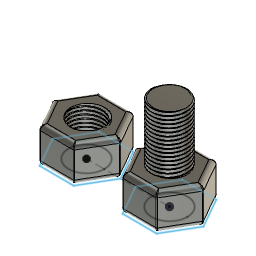
Nuts_and_Bolts (Autodesk Fusion 360 design; units mm, degrees)
Autodesk Fusion 360 part; units mm, degrees
sketch "Sketch1" plane through (0, 0, 0) normal (0, 0, 1) x (1, 0, 0)
sketch "Sketch3" plane through (0, 0, 0) normal (0, 0, 1) x (1, 0, 0)
  line L0 (7.3002, 12.4515) -> (-7.1332, 12.5479)
  line L1 (-7.1332, 12.5479) -> (-14.4334, 0.0964)
  line L2 (-14.4334, 0.0964) -> (-7.3002, -12.4515)
  line L3 (-7.3002, -12.4515) -> (7.1332, -12.5479)
  line L4 (7.1332, -12.5479) -> (14.4334, -0.0964)
  line L5 (14.4334, -0.0964) -> (7.3002, 12.4515)
  circle A0 centre (0, 0) radius 7.5
  line L6 (0, 0) -> (-35, 0) construction
  circle A1 centre (-35, 0) radius 7.5
  line L7 (-27.6998, 12.4515) -> (-42.1332, 12.5479)
  line L8 (-27.8668, -12.5479) -> (-20.5666, -0.0964)
  line L9 (-20.5666, -0.0964) -> (-27.6998, 12.4515)
  line L10 (-42.3002, -12.4515) -> (-27.8668, -12.5479)
  line L11 (-42.1332, 12.5479) -> (-49.4334, 0.0964)
  line L12 (-49.4334, 0.0964) -> (-42.3002, -12.4515)
  point P0 (-35, 0)
  point P1 (-35, 0)
  point P2 (-35, 0)
  dimension "d3" = 25
  dimension "d4" = 15
  dimension "d5" = 25
  dimension "d6" = 15
  dimension "d7" = 35
  constraint coincident A0.centre L6.start
  constraint horizontal L6
  constraint coincident P2 P1
  measures "d3" distance of L1.end L3.end
  measures "d4" diameter of A0
  measures "d5" distance of L11.end L8.start
  measures "d6" diameter of A1
  measures "d7" distance of A0.centre P2
sketch "Sketch4" plane through (0, 0, 0) normal (0, 0, 1) x (1, 0, 0)
extrude "Extrude1" add sketch "Sketch3" along normal blind 40 contours A0 makes body 1
extrude "Extrude2" add sketch "Sketch3" along normal blind 15 bodies 1 makes body 2 at (-27.5373, -0.7468, 10)
thread "Thread1" "ISO Metric profile 15.0 M15x1.5 6H" major diameter 15.2033 minor diameter 13.5262 pitch 1.5 angle 60 modelled right hand crest width 0.4068 on face at (-27.5373, -0.7468, 10) crest through (-28.2369, 0, 0.375) on bodies 2
thread "Thread2" "ISO Metric profile 15.0 M15x1.5 6g" major diameter 14.85 minor diameter 13.1369 pitch 1.5 angle 60 modelled right hand crest width 0.2152 on face at (7.4627, -0.7468, 23.3333) crest through (7.425, 0, 14.625) on bodies 1
fillet "Fillet1" radius 2 6 edges at (-0.0835, -12.4997, 15) (-10.8668, -6.1776, 15) (-10.7833, 6.3222, 15) (0.0835, 12.4997, 15) (10.8668, 6.1776, 15) (10.7833, -6.3222, 15) on bodies 1
fillet "Fillet2" radius 2 6 edges at (-24.2167, -6.3222, 15) (-35.0835, -12.4997, 15) (-45.8668, -6.1776, 15) (-45.7833, 6.3222, 15) (-34.9165, 12.4997, 15) (-24.1332, 6.1776, 15) on bodies 2
fillet "Fillet3" radius 2 12 edges at (0.0835, 12.4997, 0) (10.8668, 6.1776, 0) (10.7833, -6.3222, 0) (-0.0835, -12.4997, 0) (-10.8668, -6.1776, 0) (-10.7833, 6.3222, 0) (-34.9165, 12.4997, 0) (-24.1332, 6.1776, 0) (-24.2167, -6.3222, 0) (-35.0835, -12.4997, 0) (-45.8668, -6.1776, 0) (-45.7833, 6.3222, 0) on bodies 1 2
fillet "Fillet4" radius 0.5 36 edges at (6.799, -11.9599, 0.5858) (7.1332, -12.5479, 7.5) (6.799, -11.9599, 14.4142) (-6.9581, -11.868, 0.5858) (-7.3002, -12.4515, 7.5) (-6.9581, -11.868, 14.4142) (-13.757, 0.0919, 0.5858) (-14.4334, 0.0964, 7.5) (-13.757, 0.0919, 14.4142) (13.757, -0.0919, 0.5858) (14.4334, -0.0964, 7.5) (13.757, -0.0919, 14.4142) (6.9581, 11.868, 14.4142) (7.3002, 12.4515, 7.5) (6.9581, 11.868, 0.5858) (-6.799, 11.9599, 14.4142) (-7.1332, 12.5479, 7.5) (-6.799, 11.9599, 0.5858) (-28.0419, 11.868, 14.4142) (-27.6998, 12.4515, 7.5) (-28.0419, 11.868, 0.5858) (-41.799, 11.9599, 14.4142) (-42.1332, 12.5479, 7.5) (-41.799, 11.9599, 0.5858) (-48.757, 0.0919, 14.4142) (-49.4334, 0.0964, 7.5) (-48.757, 0.0919, 0.5858) (-21.243, -0.0919, 14.4142) (-20.5666, -0.0964, 7.5) (-21.243, -0.0919, 0.5858) (-28.201, -11.9599, 14.4142) (-27.8668, -12.5479, 7.5) (-28.201, -11.9599, 0.5858) (-41.9581, -11.868, 14.4142) (-42.3002, -12.4515, 7.5) (-41.9581, -11.868, 0.5858) on bodies 1 2
